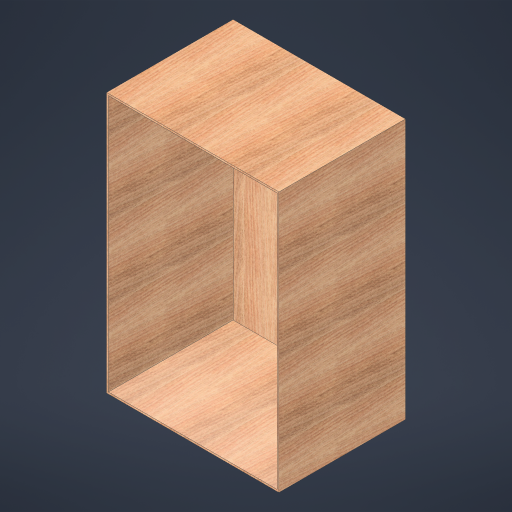
# Autodesk Inventor part: old battery cart
Saved by Autodesk Inventor 2023.4 (Build 274418000, 418)
## iProperties
Created: 2025-03-02
Part Number: old battery cart
Material: Wood (Birch)
Document SubType Name: Modeling
Designer: brand
Density: 0.55 g/cm^3
Appearance: Birch - Natural Polished
Author: brand
Autodesk Inventor part; units mm, degrees
ref_plane "YZ Plane" through (0, 0, 0) normal (1, 0, 0) x (0, 1, 0)
ref_plane "XZ Plane" through (0, 0, 0) normal (0, 1, 0) x (-1, 0, 0)
ref_plane "XY Plane" through (0, 0, 0) normal (0, 0, 1) x (1, 0, 0)
sketch "Sketch1" plane through (0, 0, 0) normal (0, 0, 1) x (1, 0, 0)
  line L0 (-292.1, -444.5) -> (292.1, -444.5)
  line L1 (292.1, -444.5) -> (292.1, 444.5)
  line L2 (292.1, 444.5) -> (-292.1, 444.5)
  line L3 (-292.1, 444.5) -> (-292.1, -444.5)
  line L4 (-292.1, -444.5) -> (292.1, 444.5) construction
  line L5 (292.1, -444.5) -> (-292.1, 444.5) construction
  line L6 (-298.45, 450.85) -> (298.45, 450.85)
  line L7 (298.45, 450.85) -> (298.45, -450.85)
  line L8 (298.45, -450.85) -> (-298.45, -450.85)
  line L9 (-298.45, -450.85) -> (-298.45, 450.85)
  point P0 (0, 0)
  dimension "d0" = 584.2
  dimension "d1" = 889
  dimension "d4" = 6.35
  constraints: 20 end point, 4 parallel, 2 midpoint, 2 perpendicular, 1 horizontal, 3 other
  measures "d0" distance of L2.end L1.end
  measures "d1" distance of L1.end L0.end
  measures "d4" distance between parallel lines of L2 L6
extrude "Extrusion1" add sketch "Sketch1" against normal blind 438.15 contours L3 L2 L1 L0 | L6 L7 L8 L9
extrude "Extrusion2" cut sketch "Sketch1" against normal blind 431.8 contours L3 L2 L1 L0
body "Solid1"
